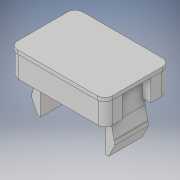
# Autodesk Inventor part: Toyota Yaris Aux Cap
Saved by Autodesk Inventor 2018 (Build 220112000, 112)
## iProperties
Created: 2017-10-18
Part Number: Toyota Yaris Aux Cap
Material: Generic
Document SubType Name: Modeling
Designer: xdlea
Density: 1 g/cm^3
Appearance: Default
Author: xdlea
Autodesk Inventor part; units mm, degrees
ref_plane "YZ Plane" through (0, 0, 0) normal (1, 0, 0) x (0, 1, 0)
ref_plane "XZ Plane" through (0, 0, 0) normal (0, 1, 0) x (-1, 0, 0)
ref_plane "XY Plane" through (0, 0, 0) normal (0, 0, 1) x (1, 0, 0)
sketch "Sketch - Main Body" plane through (0, 0, 0) normal (0, 1, 0) x (-1, 0, 0)
  line L0 (-16.925, 11.65) -> (16.925, 11.65)
  line L1 (16.925, 11.65) -> (16.925, -11.65)
  line L2 (16.925, -11.65) -> (-16.925, -11.65)
  line L3 (-16.925, -11.65) -> (-16.925, 11.65)
  line L4 (-16.925, 11.65) -> (16.925, -11.65) construction
  line L5 (16.925, 11.65) -> (-16.925, -11.65) construction
  line L6 (-16.65, 11.25) -> (16.65, 11.25)
  line L7 (16.65, -11.25) -> (-16.65, -11.25)
  line L8 (-16.65, 11.25) -> (16.65, -11.25) construction
  line L9 (16.65, 11.25) -> (-16.65, -11.25) construction
  line L10 (16.65, 5) -> (12.65, 5)
  line L11 (12.65, 5) -> (12.65, -5)
  line L12 (12.65, -5) -> (16.65, -5)
  line L13 (-16.65, 5) -> (-12.65, 5)
  line L14 (-12.65, 5) -> (-12.65, -5)
  line L15 (-12.65, -5) -> (-16.65, -5)
  line L16 (16.65, 11.25) -> (16.65, 5)
  line L17 (16.65, -5) -> (16.65, -11.25)
  line L18 (-16.65, -11.25) -> (-16.65, -5)
  line L19 (-16.65, 5) -> (-16.65, 11.25)
  line L20 (-15.65, -10.25) -> (15.65, -10.25)
  line L21 (15.65, -10.25) -> (15.65, -6)
  line L22 (15.65, -6) -> (11.65, -6)
  line L23 (11.65, -6) -> (11.65, 6)
  line L24 (11.65, 6) -> (15.65, 6)
  line L25 (15.65, 6) -> (15.65, 10.25)
  line L26 (15.65, 10.25) -> (-15.65, 10.25)
  line L27 (-15.65, 10.25) -> (-15.65, 6)
  line L28 (-15.65, 6) -> (-11.65, 6)
  line L29 (-11.65, 6) -> (-11.65, -6)
  line L30 (-11.65, -6) -> (-15.65, -6)
  line L31 (-15.65, -6) -> (-15.65, -10.25)
  circle A0 centre (-14.1819, 8.9069) radius 2.7431
  circle A1 centre (14.1819, -8.9069) radius 2.7431
  point P0 (0, 0)
  point P1 (12.65, 0)
  point P2 (0, 0)
  dimension "d0" = 33.85
  dimension "d1" = 23.3
  dimension "d2" = 33.3
  dimension "d3" = 22.5
  dimension "d4" = 10
  dimension "d5" = 4
  dimension "d6" = 1
  dimension "d26" = 38.98
  dimension "d27" = 5.4863
  constraints: 64 end point, 21 perpendicular, 12 parallel, 9 collinear, 6 midpoint, 4 tangent, 3 horizontal, 2 centre point, 1 equal radius, 1 horizontal alignment, 11 other
  measures "d0" distance of L1.end L2.end
  measures "d1" distance of L0.end L1.end
  measures "d2" distance of L7.start L7.end
  measures "d3" distance of L6.end L7.start
  measures "d4" distance of L10.end L11.end
  measures "d5" distance of L11.end L12.end
  measures "d6" distance between parallel lines of L7 L20
  measures "d27" diameter of A0
extrude "Extrusion1" add sketch "Sketch - Main Body" against normal blind 1.35
extrude "Extrusion2" add sketch "Sketch - Main Body" along normal blind 8 contours A0 L26 L27 L19 L6 | L6 L16 L10 L11 L12 L17 A1 L21 L22 L23 L24 L25 L26 A0 | A0 L19 L6 | A0 L27 L28 L29 L30 L31 L20 A1 L7 L18 L15 L14 L13 L19 | L17 A1 L7 L20 L21 | L17 L7 A1
sketch "Sketch2" plane through (0, 0, 0) normal (0, 0, 1) x (1, 0, 0)
  line L0 (-11.65, 0) -> (-11.65, 21)
  line L1 (-15.65, 0) -> (-11.65, 0) projected
  line L2 (-11.65, 0) -> (-12.8159, 0)
  line L3 (-12.65, 0) -> (-16.65, 0) projected
  line L4 (-12.65, 0) -> (-12.65, 1.5)
  line L5 (-12.65, 0) -> (-12.65, 8) projected
  line L6 (-12.65, 1.5) -> (-13.65, 3.2321)
  line L7 (-13.65, 3.2321) -> (-13.65, 10.5)
  line L8 (-13.65, 10.5) -> (-14.55, 15)
  line L9 (-14.55, 15) -> (-14.8, 15)
  line L10 (-14.8, 15) -> (-14.8, 16.5)
  line L11 (-14.8, 16.5) -> (-12.65, 21)
  line L12 (-12.65, 21) -> (-11.65, 21)
  line L13 (-16.65, 0) -> (-16.65, 8) projected
  point P0 (0, 0)
  dimension "d11" = 1.5
  dimension "d12" = 1.5
  dimension "d13" = 3
  dimension "d14" = 30
  dimension "d15" = 3.15
  dimension "d16" = 1
  dimension "d17" = 4.5
  dimension "d18" = 21
  dimension "d19" = 10.5
  dimension "d20" = 0.25
  constraints: 20 end point, 2 vertical, 1 collinear, 1 horizontal, 1 parallel, 1 perpendicular, 1 point on line
  measures "d11" distance of L9.end L10.end
  measures "d12" distance of L3.start L4.end
  measures "d13" distance between parallel lines of L13 L7
  measures "d14" angle of L7 L6
  measures "d15" distance between parallel lines of L0 L10
  measures "d16" distance of L11.end L0.end
  measures "d17" distance from line of L12 L10.end
  measures "d18" distance of L0.start L0.end
  measures "d19" vertical distance of L0.start L7.end
  measures "d20" distance of L8.end L9.end
extrude "Extrusion3" add sketch "Sketch2" along normal mid plane 12
mirror "Mirror1" about plane through (0, 0, 0) normal (1, 0, 0) of "Extrusion3"
fillet "Fillet1" radius 2.5 4 edges at (16.65, 4, 11.25) (16.65, 4, -11.25) (-16.65, 4, -11.25) (-16.65, 4, 11.25)
fillet "Fillet2" radius 2.75 4 edges at (16.925, -0.675, 11.65) (-16.925, -0.675, 11.65) (16.925, -0.675, -11.65) (-16.925, -0.675, -11.65)
body "Solid1"
